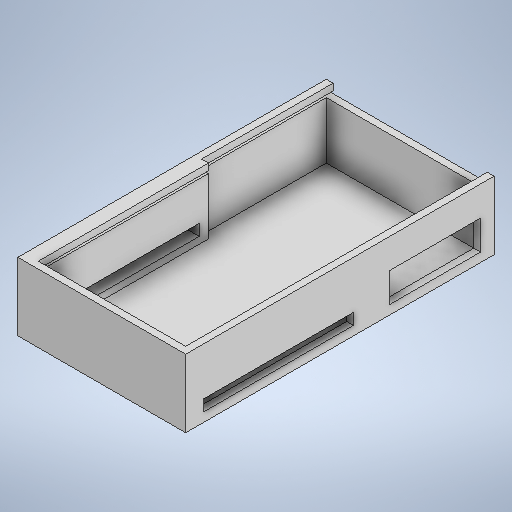
# Autodesk Inventor part: ESP 32 a&b gabung test 4
Saved by Autodesk Inventor 2025.3 (Build 293356000, 356)
## iProperties
Created: 2026-02-06
Part Number: ESP 32 a&b gabung test 4
Material: Generic
Document SubType Name: Modeling
Designer: Maulana
Density: 1 g/cm^3
Appearance: Default
Author: Maulana
Autodesk Inventor part; units mm, degrees
sketch "Sketch1" plane through (0, 0, 0) normal (0, 1, 0) x (-1, 0, 0)
  line L0 (0, 0) -> (68, 0)
  line L1 (68, -75) -> (68, -130)
  line L2 (68, -130) -> (0, -130)
  line L3 (0, -130) -> (0, 0)
  line L4 (68, 0) -> (65, 0)
  line L5 (65, 0) -> (65, -75)
  line L6 (65, -75) -> (68, -75)
  line L7 (0, 0) -> (0, 1)
  line L8 (0, 1) -> (69, 1)
  line L9 (69, 1) -> (69, -131)
  line L10 (69, -131) -> (-1, -131)
  line L11 (-1, -131) -> (-1, 1)
  line L12 (-1, 1) -> (0, 1)
  dimension "d0" = 68
  dimension "d1" = 130
  dimension "d2" = 3
  dimension "d3" = 75
  dimension "d4" = 1
  dimension "d5" = 69
  dimension "d6" = 132
  dimension "d7" = 70
  constraints: 26 end point, 8 perpendicular, 2 point on line, 1 horizontal, 1 parallel, 1 vertical
  measures "d0" distance of L0.start L0.end
  measures "d1" distance of L0.end L1.end
  measures "d2" distance of L0.end L4.end
  measures "d3" distance of L4.end L5.end
  measures "d4" distance of L0.start L7.end
  measures "d5" distance of L7.end L8.end
  measures "d6" distance of L8.end L9.end
  measures "d7" distance of L9.end L10.end
extrude "Extrusion1" add sketch "Sketch1" along normal blind 30
sketch "Sketch2" plane through (0, 0, 0) normal (0, -1, 0) x (1, 0, 0)
  line L0 (0, 0) -> (-65, 0) projected
  line L1 (-68, -75) -> (-68, -130) projected
  line L2 (0, 0) -> (-68, 0)
  line L3 (-68, 0) -> (-68, -130)
  line L4 (-68, -130) -> (0, -130)
  line L5 (0, -130) -> (0, 0)
  constraints: 8 end point, 2 parallel, 1 horizontal, 1 perpendicular
extrude "Extrusion2" add sketch "Sketch2" against normal blind 1
sketch "Sketch3" plane through (1, 0, 1) normal (1, 0, 0) x (0, 0, -1)
  line L0 (131, 1) -> (1, 1) projected
  line L1 (1, 1) -> (1, 6)
  line L2 (1, 1) -> (1, 30) projected
  line L3 (1, 6) -> (1, 1)
  line L4 (1, 6) -> (6, 6)
  line L5 (6, 9.0023) -> (72, 9.0023)
  line L6 (72, 9.0023) -> (72, 4.0023)
  line L7 (72, 4.0023) -> (6, 4.0023)
  line L8 (6, 4.0023) -> (6, 9.0023)
  line L9 (6, 1) -> (6, 4)
  point P0 (1, 0)
  dimension "d12" = 5
  dimension "d13" = 5
  dimension "d14" = 5
  dimension "d15" = 66
  dimension "d23" = 3
  constraints: 16 end point, 2 horizontal, 2 parallel, 1 collinear, 1 perpendicular, 1 point on line
  measures "d12" distance of L0.end L1.end
  measures "d13" distance of L1.end L0.end
  measures "d14" distance of L4.end L1.end
  measures "d15" distance of L6.end L7.end
  measures "d23" distance of L9.start L9.end
extrude "Extrusion3" cut sketch "Sketch3" along normal blind 34.75 and the other way blind 4
ref_plane "Work Plane1" through (-34, 30, -130) normal (-1, 0, 0) x (0, 0, 1)
mirror "Mirror1" about plane through (-34, 30, -130) normal (-1, 0, 0) of "Extrusion3"
sketch "Sketch4" plane through (1, 0, 1) normal (1, 0, 0) x (0, 0, -1)
  line L0 (131, 1) -> (131, 30) projected
  line L1 (131, 1) -> (128, 1)
  line L2 (76, 1) -> (131, 1) projected
  line L3 (128, 3.992) -> (128, 16.992)
  line L4 (128, 16.992) -> (88, 16.992)
  line L5 (88, 16.992) -> (88, 3.992)
  line L6 (88, 3.992) -> (128, 3.992)
  line L7 (132, 0) -> (0, 0) projected
  line L8 (88, 1) -> (88, 4)
  point P0 (1, 0)
  dimension "d18" = 3
  dimension "d19" = 13
  dimension "d20" = 40
  dimension "d24" = 3
  constraints: 12 end point, 3 perpendicular, 1 parallel
  measures "d18" distance of L1.end L0.start
  measures "d19" distance of L3.start L3.end
  measures "d20" distance of L3.end L4.end
  measures "d24" distance of L8.start L8.end
extrude "Extrusion4" cut sketch "Sketch4" against normal blind 5
sketch "Sketch5" plane through (-69, 0, 1) normal (0, 0, 1) x (1, 0, 0)
  line L0 (70, 0) -> (70, 30) projected
  line L1 (0, 0) -> (70, 0)
  line L2 (70, 0) -> (70, 30)
  line L3 (70, 30) -> (0, 30)
  line L4 (0, 30) -> (0, 0)
  point P0 (69, 0)
  constraints: 8 end point, 2 parallel, 1 horizontal, 1 perpendicular
extrude "Extrusion5" add sketch "Sketch5" along normal blind 2
ref_plane "Work Plane2" through (0, 30, -65) normal (0, 0, -1) x (-1, 0, 0)
mirror "Mirror2" about plane through (0, 30, -65) normal (0, 0, -1) of "Extrusion5"
sketch "Sketch6" plane through (1, 0, 3) normal (1, 0, 0) x (0, 0, -1)
  line L0 (0, 0) -> (0, 30) projected
  line L1 (0, 0) -> (136, 0) projected
  line L2 (0, 30) -> (136, 30)
  line L3 (136, 30) -> (136, 0)
  line L4 (136, 0) -> (0, 0)
  line L5 (0, 0) -> (0, 30)
  point P0 (3, 0)
  constraints: 8 end point, 2 parallel, 1 horizontal, 1 perpendicular
extrude "Extrusion6" add sketch "Sketch6" along normal blind 2
ref_plane "Work Plane3" through (-34, 30, -75) normal (1, 0, 0) x (0, 0, -1)
mirror "Mirror3" about plane through (-34, 30, -75) normal (1, 0, 0) of "Extrusion6"
sketch "Sketch7" plane through (-71, 0, -133) normal (-1, 0, 0) x (0, 0, 1)
  line L0 (62, 9.0023) -> (128, 9.0023) projected
  line L1 (128, 4.0023) -> (62, 4.0023) projected
  line L2 (62, 9.0023) -> (128, 9.0023)
  line L3 (128, 9.0023) -> (128, 4.0023)
  line L4 (128, 4.0023) -> (62, 4.0023)
  line L5 (62, 4.0023) -> (62, 9.0023)
  point P0 (133, 0)
  point P1 (62, 4.0023)
  constraints: 8 end point, 2 parallel, 1 horizontal, 1 perpendicular
extrude "Extrusion7" cut sketch "Sketch7" against normal blind 34.75
mirror "Mirror4" about plane through (-34, 30, -130) normal (-1, 0, 0) of "Extrusion7"
sketch "Sketch8" plane through (3, 0, 3) normal (1, 0, 0) x (0, 0, -1)
  line L0 (130, 16.992) -> (90, 16.992) projected
  line L1 (90, 3.992) -> (130, 3.992) projected
  line L2 (90, 16.992) -> (130, 16.992)
  line L3 (130, 16.992) -> (130, 3.992)
  line L4 (130, 3.992) -> (90, 3.992)
  line L5 (90, 3.992) -> (90, 16.992)
  point P0 (3, 0)
  constraints: 8 end point, 2 parallel, 1 horizontal, 1 perpendicular
extrude "Extrusion8" cut sketch "Sketch8" against normal blind 34.75
sketch "Sketch9" plane through (3, 0, -133) normal (0, 0, -1) x (-1, 0, 0)
  line L0 (71, 1) -> (71, 30) projected
  line L1 (71, 30) -> (71, 27)
  line L2 (71, 1) -> (71, 30) projected
  line L3 (71, 27) -> (72.5, 27)
  line L4 (74, 0) -> (74, 30) projected
  line L5 (74, 30) -> (0, 30) projected
  line L6 (3, 30) -> (3, 27)
  line L7 (3, 27) -> (1.5, 27)
  line L8 (72.5, 27) -> (1.5, 27)
  line L9 (1.5, 27) -> (1.5, 26)
  line L10 (1.5, 26) -> (72.5, 26)
  line L11 (72.5, 26) -> (72.5, 27)
  point P0 (3, 0)
  dimension "d35" = 3
  dimension "d36" = 1.5
  dimension "d37" = 1.5
  dimension "d38" = 1
  constraints: 16 end point, 3 perpendicular, 2 parallel, 2 point on line, 1 horizontal, 1 vertical
  measures "d35" distance of L0.end L1.end
  measures "d36" distance of L1.end L3.end
  measures "d37" distance of L6.end L7.end
  measures "d38" distance of L9.end L8.end
extrude "Extrusion9" cut sketch "Sketch9" against normal blind 133 contours L3 L11 L10 L0 | L0 L10 L9 L7 L8
sketch "Sketch10" plane through (3, 0, -133) normal (0, 0, -1) x (-1, 0, 0)
  line L0 (0, 30) -> (74, 30) projected
  line L1 (71, 27) -> (3, 27) projected
  line L2 (3, 30) -> (71, 30)
  line L3 (71, 30) -> (71, 27)
  line L4 (71, 27) -> (3, 27)
  line L5 (3, 27) -> (3, 30)
  point P0 (3, 0)
  constraints: 8 end point, 2 parallel, 1 horizontal, 1 perpendicular, 1 point on line
extrude "Extrusion10" cut sketch "Sketch10" against normal blind 3
body "Solid1"
